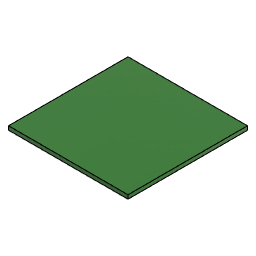
main v11 (Autodesk Fusion 360 archive; units mm, degrees)
design "pcb"
Autodesk Fusion 360 part; units mm, degrees
sketch "Sketch1" plane through (0, 0, 0) normal (0, 0, 1) x (1, 0, 0)
  line L0 (-25, 25) -> (25, 25)
  line L1 (25, 25) -> (25, -25)
  line L2 (25, -25) -> (-25, -25)
  line L3 (-25, -25) -> (-25, 25)
  dimension "d1" = 25
  dimension "d2" = 25
  dimension "d3" = 25
  dimension "d4" = 25
  constraint horizontal L0
  constraint vertical L1
  constraint horizontal L2
  constraint vertical L3
  measures "d1" distance of origin L1
  measures "d2" distance of origin L3
  measures "d3" distance of origin L0
  measures "d4" distance of origin L2
extrude "Extrude1" add sketch "Sketch1" along normal blind 1.6
equation "d2 = d1"
equation "d3 = d1"
equation "d4 = d1"

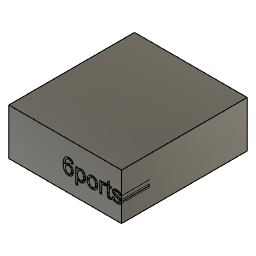
design "SF-801-8-port-10/100-module"
Autodesk Fusion 360 part; units mm, degrees
sketch "Sketch1" plane through (0, 0, 0) normal (0, 0, 1) x (1, 0, 0)
  line L0 (-36.5, 40.7) -> (36.5, 40.7)
  line L1 (36.5, 40.7) -> (36.5, -40.7)
  line L2 (36.5, -40.7) -> (-36.5, -40.7)
  line L3 (-36.5, -40.7) -> (-36.5, 40.7)
  dimension "d1" = 40.7
  dimension "d2" = 40.7
  dimension "d3" = 36.5
  dimension "d4" = 36.5
  constraint horizontal L0
  constraint vertical L1
  constraint horizontal L2
  constraint vertical L3
  measures "d1" distance of origin L0
  measures "d2" distance of origin L2
  measures "d3" distance of origin L1
  measures "d4" distance of origin L3
extrude "Extrude1" add sketch "Sketch1" along normal blind 30
sketch "Sketch2" plane through (0, -40.7, 0) normal (0, -1, 0) x (1, 0, 0)
  line L0 (-36.5, 0) -> (36.5, 0)
  line L1 (36.5, 0) -> (36.5, 30)
  line L2 (36.5, 30) -> (-36.5, 30)
  line L3 (-36.5, 30) -> (-36.5, 0)
  line L4 (-36.5, 0) -> (36.5, 0) construction
  line L5 (36.5, 0) -> (36.5, 30) construction
  line L6 (36.5, 30) -> (-36.5, 30) construction
  line L7 (-36.5, 30) -> (-36.5, 0) construction
  dimension "d7" = 10
  text T0 "6ports" font "Arial" height 10 align right middle in box 73 x 30 at (-36.5, 0) x (1, 0) y (0, 1) spacing 1 kerned
  constraint coincident L0.end
  constraint coincident L2.end
extrude "Extrude2" cut sketch "Sketch2" against normal blind 18 text T0
equation "d1 = ( 81.4 / 2 ) * 1 mm"
equation "d2 = d1"
equation "d3 = ( 73 / 2 ) * 1 mm"
equation "d4 = d3"

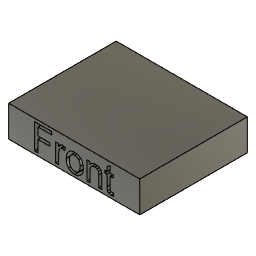
design "centerm-c33m"
Autodesk Fusion 360 part; units mm, degrees
sketch "Sketch1" plane through (0, 0, 0) normal (0, 0, 1) x (1, 0, 0)
  line L0 (-78, 64) -> (78, 64)
  line L1 (78, 64) -> (78, -64)
  line L2 (78, -64) -> (-78, -64)
  line L3 (-78, -64) -> (-78, 64)
  dimension "d1" = 78
  dimension "d2" = 78
  dimension "d3" = 64
  dimension "d4" = 64
  constraint horizontal L0
  constraint vertical L1
  constraint horizontal L2
  constraint vertical L3
  measures "d1" distance of origin L1
  measures "d2" distance of origin L3
  measures "d3" distance of origin L0
  measures "d4" distance of origin L2
extrude "Extrude1" add sketch "Sketch1" along normal blind 37
sketch "Sketch2" plane through (0, -64, 0) normal (0, -1, 0) x (1, 0, 0)
  line L0 (-78, 0) -> (78, 0)
  line L1 (78, 0) -> (78, 37)
  line L2 (78, 37) -> (-78, 37)
  line L3 (-78, 37) -> (-78, 0)
  line L4 (-78, 0) -> (78, 0) construction
  line L5 (78, 0) -> (78, 37) construction
  line L6 (78, 37) -> (-78, 37) construction
  line L7 (-78, 37) -> (-78, 0) construction
  dimension "d7" = 30
  text T0 "Front" font "Arial" height 30 align centre middle in box 156 x 37 at (-78, 0) x (1, 0) y (0, 1) spacing 1 kerned
  constraint coincident L0.end
  constraint coincident L2.end
extrude "Extrude2" cut sketch "Sketch2" against normal blind 20 text T0
equation "d1 = ( 156 / 2 ) * 1 mm"
equation "d2 = d1"
equation "d3 = ( 128 / 2 ) * 1 mm"
equation "d4 = d3"

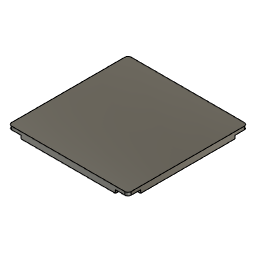
design "to-cover"
Autodesk Fusion 360 part; units mm, degrees
sketch "Sketch1" plane through (0, 0, 0) normal (0, 0, 1) x (1, 0, 0)
  line L0 (90, 95) -> (-90, 95)
  line L1 (-95, 90) -> (-95, -90)
  line L2 (-90, -95) -> (90, -95)
  line L3 (95, -90) -> (95, 90)
  arc A0 (95, 90) -> (90, 95) centre (90, 90) ccw
  arc A1 (-90, 95) -> (-95, 90) centre (-90, 90) ccw
  arc A2 (-95, -90) -> (-90, -95) centre (-90, -90) ccw
  arc A3 (90, -95) -> (95, -90) centre (90, -90) ccw
  point P0 (95, 95)
  point P1 (-95, 95)
  point P2 (95, -95)
  dimension "d1" = 190
  dimension "d2" = 190
  dimension "d3" = 95
  dimension "d4" = 95
  dimension "d5" = 5
  constraint horizontal L0
  constraint vertical L1
  constraint horizontal L2
  constraint vertical L3
  constraint coincident P0 L3
  constraint coincident P0 L0
  constraint tangent L3 A0
  constraint tangent L0 A0
  constraint coincident P1 L0
  constraint coincident P1 L1
  constraint tangent L0 A1
  constraint tangent L1 A1
  constraint equal A0 A1
  constraint tangent L1 A2
  constraint tangent L2 A2
  constraint equal A0 A2
  constraint coincident P2 L2
  constraint coincident P2 L3
  constraint tangent L2 A3
  constraint tangent L3 A3
  constraint equal A0 A3
  measures "d1" distance of P0 P1
  measures "d2" distance of P0 P2
  measures "d3" distance of origin L1
  measures "d4" distance of origin L0
  measures "d5" radius of A0
extrude "Extrude1" add sketch "Sketch1" along normal blind 5
sketch "Sketch2" plane through (0, 0, 0) normal (0, 0, -1) x (1, 0, 0)
  arc A0 (95, 90) -> (90, 95) centre (90, 90) ccw
  line L0 (90, 95) -> (-90, 95)
  arc A1 (-90, 95) -> (-95, 90) centre (-90, 90) ccw
  line L1 (-95, 90) -> (-95, -90)
  arc A2 (-95, -90) -> (-90, -95) centre (-90, -90) ccw
  line L2 (-90, -95) -> (90, -95)
  arc A3 (90, -95) -> (95, -90) centre (90, -90) ccw
  line L3 (95, -90) -> (95, 90)
  line L4 (-95, 95) -> (95, 95)
  line L5 (95, 95) -> (95, -95)
  line L6 (95, -95) -> (-95, -95)
  line L7 (-95, -95) -> (-95, 95)
  line L8 (95, -95) -> (75, -95)
  line L9 (75, -95) -> (75, -75)
  line L10 (75, -75) -> (95, -75)
  line L11 (95, -75) -> (95, -95)
  line L12 (-95, -95) -> (-75, -95)
  line L13 (-75, -95) -> (-75, -75)
  line L14 (-75, -75) -> (-95, -75)
  line L15 (-95, -75) -> (-95, -95)
  line L16 (95, 95) -> (75, 95)
  line L17 (75, 95) -> (75, 75)
  line L18 (75, 75) -> (95, 75)
  line L19 (95, 75) -> (95, 95)
  line L20 (-95, 95) -> (-75, 95)
  line L21 (-75, 95) -> (-75, 75)
  line L22 (-75, 75) -> (-95, 75)
  line L23 (-95, 75) -> (-95, 95)
  dimension "d8" = 20
  dimension "d9" = 20
  constraint horizontal L4
  constraint vertical L5
  constraint horizontal L6
  constraint vertical L7
  constraint horizontal L8
  constraint vertical L9
  constraint horizontal L10
  constraint vertical L11
  constraint horizontal L12
  constraint vertical L13
  constraint horizontal L14
  constraint vertical L15
  constraint horizontal L16
  constraint vertical L17
  constraint horizontal L18
  constraint vertical L19
  constraint horizontal L20
  constraint vertical L21
  constraint horizontal L22
  constraint vertical L23
  constraint coincident A1.end L7
  constraint coincident A3.end L5
  constraint coincident L2.end L6
  constraint coincident A0.end L4
  constraint equal L17 L21
  constraint equal L13 L21
  constraint equal L9 L21
  constraint equal L18 L22
  constraint equal L10 L22
  constraint equal L14 L22
  measures "d8" distance of L20.end L21.end
  measures "d9" distance of L21.end L22.end
extrude "Extrude2" add sketch "Sketch2" along normal blind 5 contours L0 L1 L2 L3 L4 L5 L6 L7 L9 L10 L13 L14 L17 L18 L21 L22
equation "d2 = d1"
equation "d3 = d1 / 2"
equation "d4 = d1 / 2"
